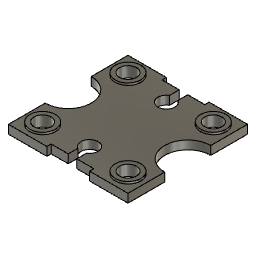
Model 19 (Autodesk Fusion 360 design; units mm, degrees)
Autodesk Fusion 360 part; units mm, degrees
sketch "Sketch1" plane through (0, 0, 0) normal (0, 0, 1) x (1, 0, 0)
  line L0 (0, 86) -> (0, 40) construction
  line L1 (0, 40) -> (40, 40) construction
  circle A0 centre (40, 40) radius 20
  circle A1 centre (40, 40) radius 30
  line L2 (0, 140) -> (280, 140) construction
  line L3 (140, 280) -> (140, 0) construction
  circle A2 centre (240, 40) radius 30
  circle A3 centre (240, 40) radius 20
  circle A4 centre (240, 240) radius 30
  circle A5 centre (240, 240) radius 20
  circle A6 centre (40, 240) radius 30
  circle A7 centre (40, 240) radius 20
  arc A8 (0, 86) -> (0, 194) centre (0, 140) ccw
  line L4 (0, 280) -> (0, 194)
  line L5 (0, 86) -> (0, 0)
  line L6 (280, 0) -> (280, 86)
  line L7 (280, 194) -> (280, 280)
  arc A9 (280, 194) -> (280, 86) centre (280, 140) ccw
  line L8 (0, 0) -> (90, 0) construction
  line L9 (90, 0) -> (90, 10)
  line L10 (90, 10) -> (120, 10)
  line L11 (160, 10) -> (190, 10)
  line L12 (190, 10) -> (190, 0)
  line L13 (140, 0) -> (140, 50) construction
  line L14 (140, 50) -> (120, 50) construction
  line L15 (140, 50) -> (160, 50) construction
  line L16 (0, 0) -> (90, 0)
  line L17 (190, 0) -> (280, 0)
  line L18 (0, 280) -> (90, 280) construction
  line L19 (90, 280) -> (90, 270)
  line L20 (90, 270) -> (120, 270)
  line L21 (160, 270) -> (190, 270)
  line L22 (190, 270) -> (190, 280)
  line L23 (140, 280) -> (140, 230) construction
  line L24 (140, 230) -> (160, 230) construction
  line L25 (140, 230) -> (120, 230) construction
  line L26 (280, 280) -> (190, 280)
  line L27 (90, 280) -> (0, 280)
  line L28 (160, 270) -> (150, 270)
  line L29 (120, 270) -> (130, 270)
  line L30 (130, 270) -> (130, 247.3205)
  line L31 (150, 270) -> (150, 247.3205)
  arc A10 (130, 247.3205) -> (150, 247.3205) centre (140, 230) ccw
  line L32 (120, 10) -> (130, 10)
  line L33 (160, 10) -> (150, 10)
  line L34 (150, 10) -> (150, 32.6795)
  line L35 (130, 10) -> (130, 32.6795)
  arc A11 (150, 32.6795) -> (130, 32.6795) centre (140, 50) ccw
  point P0 (140, 140)
  dimension "d1" = 280
  dimension "d2" = 280
  dimension "d3" = 100
  dimension "d4" = 40
  dimension "d7" = 40
  dimension "d8" = 60
  dimension "d10" = 360
  dimension "d11" = 108
  dimension "d12" = 108
  dimension "d13" = 90
  dimension "d14" = 10
  dimension "d17" = 10
  dimension "d18" = 50
  dimension "d19" = 40
  dimension "d20" = 90
  dimension "d21" = 10
  dimension "d22" = 50
  dimension "d23" = 40
  dimension "d25" = 10
  dimension "d26" = 10
  dimension "d27" = 10
  dimension "d28" = 10
  constraint horizontal L16
  constraint vertical L6
  constraint horizontal L26
  constraint vertical L4
  constraint coincident L5.end L8.start
  constraint parallel L0 L4
  constraint perpendicular L1 L4
  constraint coincident L1.end A0.centre
  constraint concentric A0 A1
  constraint midpoint L3 P0
  constraint coincident L2.start A8.centre
  constraint coincident L2.end A9.centre
  constraint coincident L0.start L4
  constraint collinear L4 L5
  constraint coincident L2.start L4
  constraint collinear L6 L7
  constraint perpendicular L3 L8
  constraint perpendicular L8 L9
  constraint perpendicular L9 L10
  constraint perpendicular L3 L11
  constraint perpendicular L12 L16
  constraint perpendicular L10 L13
  constraint coincident L13.end L14.start
  constraint perpendicular L3 L14
  constraint perpendicular L3 L15
  constraint collinear L16 L17
  constraint perpendicular L3 L18
  constraint perpendicular L18 L19
  constraint perpendicular L3 L20
  constraint perpendicular L3 L21
  constraint perpendicular L22 L26
  constraint perpendicular L21 L23
  constraint coincident L23.end L24.start
  constraint perpendicular L23 L24
  constraint perpendicular L23 L25
  constraint collinear L26 L27
  constraint coincident L25.end A10
  constraint coincident L24.end A10
  constraint coincident L14.end A11
  constraint coincident L15.end A11
  constraint parallel L21 L28
  constraint perpendicular L23 L29
  constraint perpendicular L29 L30
  constraint perpendicular L28 L31
  constraint perpendicular L33 L34
  constraint perpendicular L32 L35
  measures "d1" distance of L5.end L6.start
  measures "d2" distance of L5.end L4.start
  measures "d3" distance of L2.start L0.end
  measures "d4" distance of L0.end L1.end
  measures "d7" diameter of A0
  measures "d8" diameter of A1
  measures "d11" diameter of A8
  measures "d12" diameter of A9
  measures "d13" distance of L5.end L8.end
  measures "d14" distance of L8.end L9.end
  measures "d17" distance of L11.end L12.end
  measures "d18" distance of L3.end L13.end
  measures "d19" diameter of A11
  measures "d20" distance of L4.start L18.end
  measures "d21" distance of L18.end L19.end
  measures "d22" distance of L3.start L23.end
  measures "d23" diameter of A10
  measures "d25" distance of L21.start L28.end
  measures "d26" distance of L20.end L29.end
  measures "d27" distance of L10.end L32.end
  measures "d28" distance of L11.start L33.end
extrude "Extrude1" add sketch "Sketch1" along normal blind 20 contours A8 L4 L5 L6 L7 A9 L9 L10 L11 L12 L16 L17 L19 L20 L21 L22 L26 L27 L28 L29 L30 L31 A10 L32 L33 L34 L35 A11
extrude "Extrude2" add sketch "Sketch1" along normal blind 25 contours A1 | A2 | A4 | A6
ref_plane "WorkPlane1" through (54, 140, 13.2295) normal (-1, 0, 0) x (0, 1, 0)
sketch "Sketch2" plane through (54, 140, 13.2295) normal (-1, 0, 0) x (0, 1, 0)
  line L0 (45, 10) -> (-45, 10) construction
  line L1 (-45, 10) -> (-45, -5) construction
  line L2 (-45, -5) -> (45, -5) construction
  line L3 (45, -5) -> (45, 10) construction
  text T0 "enes şahin" font "Arial" height 5 align centre middle in box 90 x 15 at (45, 10) x (-1, 0) y (0, -1) spacing 1
extrude "Extrude3" add sketch "Sketch2" along normal blind 3 text T0
